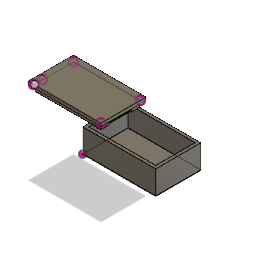
RombaIrBox (Autodesk Fusion 360 design; units mm, degrees)
Autodesk Fusion 360 part; units mm, degrees
note: some values were not read from the file. Set by a fixed rule: which sketch regions a step uses.
sketch "Base" plane through (0, 0, 0) normal (0, 1, 0) x (1, 0, 0) in component "Top"
  line L0 (0, 0) -> (37, 0)
  line L1 (37, 0) -> (37, 23)
  line L2 (37, 23) -> (0, 23)
  line L3 (0, 23) -> (0, 0)
  dimension "d6" = 37
  dimension "d7" = 23
  constraint horizontal L0
  constraint vertical L1
  constraint horizontal L2
  constraint vertical L3
  constraint coincident L0.start L3.end
  measures "d6" distance of L0.start L0.end
  measures "d7" distance of L0.start L2.end
extrude "Extrude1" add sketch "Base" along normal blind 12 makes body 1 in component "Top"
shell "Shell1" thickness 1.5 removed faces 1 at (12.3333, 12, -15.3333) on bodies 1 in component "Top"
sketch "Knob" plane through (1.5, 0, 0) normal (1, 0, 0) x (0, 0, -1) in component "Top"
  line L0 (21.5, 12) -> (1.5, 12)
  line L1 (1.5, 1.5) -> (21.5, 1.5)
  line L2 (5.75, 12) -> (17.25, 12)
  line L3 (17.25, 12) -> (17.25, 9)
  line L4 (17.25, 9) -> (5.75, 9)
  line L5 (5.75, 9) -> (5.75, 12)
  line L6 (11.5, 12) -> (11.5, 9) construction
  line L7 (21.5, 1.5) -> (21.5, 12)
  line L8 (1.5, 12) -> (1.5, 1.5)
  dimension "d12" = 11.5
  dimension "d13" = 3
  constraint horizontal L2
  constraint vertical L3
  constraint horizontal L4
  constraint vertical L5
  constraint coincident L0 L2.start
  constraint midpoint L0 L6.start
  constraint midpoint L4 L6.end
  constraint vertical L6
  measures "d12" distance of L3.end L4.end
  measures "d13" distance of L2.end L3.end
extrude "Extrude2" add sketch "Knob" along normal blind 3 draft -45 contours L0 L2 L3 L4 L5 bodies 1 in component "Top"
ref_plane "WorkPlane2" through (18.5, 6, -11.5) normal (-1, 0, 0) x (0, 0, 1) in component "Top"
mirror "Mirror1" about plane through (18.5, 6, -11.5) normal (-1, 0, 0) of "Extrude2" in component "Top"
sketch "Top" plane through (0, 12, 0) normal (0, 1, 0) x (-1, 0, 0) in component "Base"
  line L0 (-37, 0) -> (-37, -23)
  line L1 (-37, -23) -> (0, -23)
  line L2 (0, -23) -> (0, 0)
  line L3 (0, 0) -> (-37, 0)
  line L4 (-35.5, -5.75) -> (-35.5, -1.5)
  line L5 (-35.5, -1.5) -> (-1.5, -1.5)
  line L6 (-1.5, -1.5) -> (-1.5, -5.75)
  line L7 (-1.5, -5.75) -> (-1.5, -17.25)
  line L8 (-1.5, -17.25) -> (-1.5, -21.5)
  line L9 (-1.5, -21.5) -> (-35.5, -21.5)
  line L10 (-35.5, -17.25) -> (-35.5, -5.75)
  line L11 (-35.5, -21.5) -> (-35.5, -17.25)
extrude "Extrude1'" add sketch "Top" along normal blind 1.5 separate body contours L0 L1 L2 L3 | L4 L5 L6 L7 L8 L9 L10 L11 makes body 2 in component "Base"
sketch "Lip" plane through (0, 12, 0) normal (0, -1, 0) x (1, 0, 0) in component "Base"
  line L0 (37, 0) -> (0, 0)
  line L1 (0, 0) -> (0, -23)
  line L2 (0, -23) -> (37, -23)
  line L3 (37, -23) -> (37, 0)
  line L4 (35.3, -21.3) -> (35.3, -1.7)
  line L5 (35.3, -1.7) -> (1.7, -1.7)
  line L6 (1.7, -1.6987) -> (1.7, -21.3)
  line L7 (1.7, -21.3) -> (35.3, -21.3)
  line L8 (35.5, -1.5) -> (1.5, -1.5)
  line L9 (1.5, -1.5) -> (1.5, -5.75)
  line L10 (35.5, -21.5) -> (1.5, -21.5)
  constraint parallel L3 L4
  constraint parallel L0 L5
  constraint parallel L1 L6
  constraint parallel L2 L7
extrude "Extrude2'" add sketch "Lip" along normal blind 3 contours L4 L5 L6 L7 bodies 2 in component "Base"
extrude "Extrude3" cut sketch "Knob" along normal blind 3 draft -45 from surface at 0.2 contours L0 L2 L3 L4 L5 bodies 2 in component "Base"
mirror "Mirror1'" about plane through (18.5, 6, -11.5) normal (-1, 0, 0) of "Extrude3" in component "Base"
shell "Shell1'" thickness 1.5 removed faces 1 at (12.9, 9, -9.5833) on bodies 2 in component "Base"
chamfer "Chamfer1" distance 0.6 angle 45 2 edges at (1.7, 9, -11.5) (35.3, 9, -11.5) on bodies 2 in component "Base"
sketch "Sketch6" plane through (0, 25.0225, 0) normal (0, -1, 0) x (1, 0, 0)
  line L0 (24.5355, 19.009) -> (25.1355, 19.609)
  line L1 (25.1355, 19.609) -> (25.1355, 23.659)
  line L2 (25.1355, 23.659) -> (-8.4645, 23.659)
  line L3 (-8.4645, 23.659) -> (-8.4645, 19.609)
  line L4 (-8.4645, 19.609) -> (-7.8645, 19.009)
  line L5 (-7.8645, 19.009) -> (-7.8645, 8.709)
  line L6 (-7.8645, 8.709) -> (-8.4645, 8.109)
  line L7 (-8.4645, 8.109) -> (-8.4645, 4.059)
  line L8 (-8.4645, 4.059) -> (25.1355, 4.059)
  line L9 (25.1355, 8.109) -> (24.5355, 8.709)
  line L10 (24.5355, 8.709) -> (24.5355, 19.009)
  line L11 (23.6355, 5.559) -> (-6.9645, 5.559)
  line L12 (-6.9645, 5.559) -> (-6.9645, 7.4877)
  line L13 (-6.9645, 7.4877) -> (-6.3432, 8.109)
  line L14 (-6.3432, 8.109) -> (-6.3432, 19.609)
  line L15 (-6.3432, 19.609) -> (-6.9645, 20.2303)
  line L16 (-6.9645, 20.2303) -> (-6.9645, 22.159)
  line L17 (-6.9645, 22.159) -> (23.6355, 22.159)
  line L18 (23.6355, 22.159) -> (23.6355, 20.2303)
  line L19 (23.6355, 20.2303) -> (23.0142, 19.609)
  line L20 (23.0142, 19.609) -> (23.0142, 8.109)
  line L21 (23.0142, 8.109) -> (23.6355, 7.4877)
  line L22 (23.6355, 7.4877) -> (23.6355, 5.559)
  line L23 (-1.4645, 5.559) -> (18.1355, 5.559)
  line L24 (18.1355, 5.559) -> (18.1355, 4.059)
  line L25 (18.1355, 4.059) -> (-1.4645, 4.059)
  line L26 (-1.4645, 4.059) -> (-1.4645, 5.559)
  line L27 (-8.4645, 23.6603) -> (-8.4645, 4.059)
  line L28 (25.1355, 4.059) -> (25.1355, 23.659)
  line L29 (25.1355, 4.059) -> (25.1355, 8.109)
  dimension "d58" = 7
  constraint horizontal L23
  constraint vertical L24
  constraint horizontal L25
  constraint vertical L26
  constraint coincident L8 L24.end
  constraint coincident L11 L23.start
  measures "d58" distance of L24 L28
extrude "Extrude6" cut sketch "Sketch6" against normal blind 3 contours L8 L11 L23 L24 L25 L26 sketch seen with x (1, 0, 0) y (0, 1, 0) z (0, 0, 1) at (10.1645, -16.0225, -25.359) bodies 2 in component "Base"
component "Enclosure" placed x (1, 0, 0) y (0, 1, 0) z (0, 0, 1) at (0, 0, 0)
component "Top" placed x (1, 0, 0) y (0, 1, 0) z (0, 0, 1) at (-7.7688, -14.0093, 0) in component "Enclosure"
component "Base" placed x (1, 0, 0) y (0, 1, 0) z (0, 0, 1) at (-10.1645, 16.0225, 25.359) in component "Enclosure"
equation "Width = 23 mm"
equation "length = 37 mm"
equation "heigth = 12 mm"
equation "shell = 1.5 mm"
equation "gap = 0.2 mm"
equation "d6 = length"
equation "d7 = Width"
equation "d8 = heigth"
equation "d11 = shell"
equation "d12 = Width / 2"
equation "d13 = shell * 2"
equation "d17 = shell"
equation "d20 = shell * 2"
equation "d23 = shell * 2"
equation "d26 = shell"
